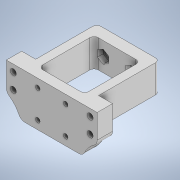
# Autodesk Inventor part: Zcarriage
Saved by Autodesk Inventor 2022 (Build 260153000, 153)
## iProperties
Created: 2022-02-20
Part Number: Zcarriage
Material: Genérico
Document SubType Name: Modeling
Designer: JK
Density: 1 g/cm^3
Appearance: Valor por defecto
Author: JK
Autodesk Inventor part; units mm, degrees
ref_plane "YZ Plane" through (0, 0, 0) normal (1, 0, 0) x (0, 1, 0)
ref_plane "XZ Plane" through (0, 0, 0) normal (0, 1, 0) x (-1, 0, 0)
ref_plane "XY Plane" through (0, 0, 0) normal (0, 0, 1) x (1, 0, 0)
sketch "Boceto1" plane through (0, 0, 0) normal (0, 1, 0) x (-1, 0, 0)
  line L0 (21.032, 35.0057) -> (-23.968, 35.0057)
  line L1 (-23.968, 35.0057) -> (-23.968, 29.0057)
  line L2 (-23.968, 29.0057) -> (21.032, 29.0057)
  line L3 (21.032, 29.0057) -> (21.032, 35.0057)
  line L4 (21.032, -10.7443) -> (-23.968, -10.7443)
  line L5 (-23.968, -10.7443) -> (-23.968, -18.7443)
  line L6 (-23.968, -18.7443) -> (21.032, -18.7443)
  line L7 (21.032, -18.7443) -> (21.032, -10.7443)
  line L8 (21.032, 29.0057) -> (21.032, -18.7443)
  line L9 (-23.968, 29.0057) -> (-23.968, -18.7443)
  line L10 (21.032, 29.0057) -> (21.032, -10.7443)
  line L11 (-23.968, 29.0057) -> (-23.968, -10.7443)
  line L12 (15.032, 29.0057) -> (15.032, -10.7443)
  line L13 (-17.968, 29.0057) -> (-17.968, -10.7443)
  point P0 (0, 0)
  dimension "d0" = 45
  dimension "d1" = 6
  dimension "d3" = 8
  dimension "d4" = 45
  dimension "d7" = 47.75
  dimension "d8" = 6
  dimension "d9" = 6
  constraints: 28 end point, 8 parallel, 6 point on line, 2 horizontal, 2 perpendicular, 1 collinear
  measures "d0" distance of L0.start L0.end
  measures "d1" distance of L2.end L0.start
  measures "d3" distance between parallel lines of L6 L4
  measures "d4" distance of L5.end L6.end
  measures "d7" distance between parallel lines of L6 L2
  measures "d8" distance of L2.end L12.start
  measures "d9" distance of L13.start L1.end
extrude "Extrusión1" add sketch "Boceto1" along normal blind 20 contours L3 L2 L1 L0 | L8 L4 L12 L2 | L2 L13 L4 L9 | L7 L6 L5 L4
sketch "Boceto2" plane through (23.968, 0, -18.7443) normal (0, 0, -1) x (-1, 0, 0)
  circle A0 centre (12.5, 10) radius 2.65
  circle A1 centre (32.5, 10) radius 2.65
  line L0 (0, 0) -> (45, 0) projected
  line L1 (45, 0) -> (45, 20) projected
  point P0 (23.968, 0)
  dimension "d10" = 5.3
  dimension "d11" = 5.3
  dimension "d12" = 20
  dimension "d14" = 10
  dimension "d17" = 12.5
  constraints: 2 centre point, 1 horizontal alignment
  measures "d10" diameter of A0
  measures "d11" diameter of A1
  measures "d12" distance of A1.centre A0.centre
  measures "d14" distance from line of A0.centre L0
  measures "d17" distance from line of L1 A1.centre
extrude "Extrusión2" cut sketch "Boceto2" against normal blind 20
fillet "Empalme1" radius 3 6 edges at (17.968, 10, -10.7443) (-15.032, 10, -10.7443) (17.968, 10, 29.0057) (-15.032, 10, 29.0057) (23.968, 10, -18.7443) (-21.032, 10, -18.7443)
sketch "Boceto3" plane through (-12.032, 0, -10.7443) normal (0, 0, 1) x (1, 0, 0)
  circle A0 centre (23.5, 10) radius 2.65 projected
  circle A1 centre (23.5, 10) radius 4.05
  circle A2 centre (3.5, 10) radius 2.65 projected
  circle A3 centre (3.5, 10) radius 4.05
  line L0 (23.5, 5.3235) -> (19.45, 7.6617)
  line L1 (19.45, 7.6617) -> (19.45, 12.3383)
  line L2 (19.45, 12.3383) -> (23.5, 14.6765)
  line L3 (23.5, 14.6765) -> (27.55, 12.3383)
  line L4 (27.55, 12.3383) -> (27.55, 7.6617)
  line L5 (27.55, 7.6617) -> (23.5, 5.3235)
  line L6 (3.5, 5.3235) -> (-0.55, 7.6617)
  line L7 (-0.55, 7.6617) -> (-0.55, 12.3383)
  line L8 (-0.55, 12.3383) -> (3.5, 14.6765)
  line L9 (3.5, 14.6765) -> (7.55, 12.3383)
  line L10 (7.55, 12.3383) -> (7.55, 7.6617)
  line L11 (7.55, 7.6617) -> (3.5, 5.3235)
  point P0 (12.032, 0)
  dimension "d19" = 8.1
  constraints: 24 end point, 4 coincident, 2 centre point, 2 tangent, 2 vertical alignment, 1 equal radius, 26 other
  measures "d19" diameter of A1
extrude "Extrusión3" cut sketch "Boceto3" along normal blind 20 and the other way blind 4 contours A0 | A1 | L4 L5 A1 | A1 L3 L4 | A1 L2 L3 | L5 L0 A1 | A1 L1 L2 | L0 L1 A1 | A2 | A3 | L10 L11 A3 | A3 L9 L10 | A3 L8 L9 | L11 L6 A3 | A3 L7 L8 | L6 L7 A3
sketch "Boceto4" plane through (0, 0, 0) normal (0, -1, 0) x (1, 0, 0)
  arc A0 (-21.032, -15.7443) -> (-18.032, -18.7443) centre (-18.032, -15.7443) ccw projected
  line L0 (20.968, -18.7443) -> (-18.032, -18.7443) projected
  arc A1 (20.968, -18.7443) -> (23.968, -15.7443) centre (20.968, -15.7443) ccw projected
  line L1 (23.968, 35.0057) -> (23.968, -15.7443) projected
  line L2 (-21.032, 35.0057) -> (23.968, 35.0057) projected
  line L3 (-21.032, -15.7443) -> (-21.032, 35.0057) projected
  arc A2 (-15.032, -7.7443) -> (-12.032, -10.7443) centre (-12.032, -7.7443) ccw projected
  line L4 (-15.032, 26.0057) -> (-15.032, -7.7443) projected
  arc A3 (-12.032, 29.0057) -> (-15.032, 26.0057) centre (-12.032, 26.0057) ccw projected
  line L5 (14.968, 29.0057) -> (-12.032, 29.0057) projected
  arc A4 (17.968, 26.0057) -> (14.968, 29.0057) centre (14.968, 26.0057) ccw projected
  line L6 (17.968, -7.7443) -> (17.968, 26.0057) projected
  arc A5 (14.968, -10.7443) -> (17.968, -7.7443) centre (14.968, -7.7443) ccw projected
  line L7 (-12.032, -10.7443) -> (14.968, -10.7443) projected
  line L8 (-21.032, 35.0057) -> (23.968, 35.0057) projected
  line L9 (23.968, 35.0057) -> (-21.032, 35.0057)
  line L10 (-21.032, 35.0057) -> (-21.032, 29.0057)
  line L11 (-21.032, 29.0057) -> (23.968, 29.0057)
  line L12 (23.968, 29.0057) -> (23.968, 35.0057)
  point P0 (0, 0)
  constraints: 8 end point, 2 parallel, 1 horizontal, 1 perpendicular, 1 point on line
extrude "Extrusión4" add sketch "Boceto4" along normal blind 12 contours L3 L2 L1 L11 L5
chamfer "Chaflán1" distance 12 angle 45 2 edges at (-16.532, 0, 29.0057) (19.468, 0, 29.0057)
sketch "Boceto5" plane through (-21.032, 20, 35.0057) normal (0, 0, 1) x (1, 0, 0)
  circle A0 centre (32.5, -6) radius 1.65
  line L0 (0, 0) -> (45, 0) projected
  line L1 (45, -32) -> (45, 0) projected
  point P0 (21.032, -20)
  dimension "d29" = 3.3
  dimension "d30" = 6
  dimension "d31" = 12.5
  constraints: 1 centre point
  measures "d29" diameter of A0
  measures "d30" distance from line of L0 A0.centre
  measures "d31" distance from line of L1 A0.centre
extrude "Extrusión5" cut sketch "Boceto5" against normal blind 21.5
pattern_linear "Patrón rectangular1" count 2 spacing 20 along (-1, 0, 0) count 2 spacing 20 along (0, -1, 0) of "Extrusión5"
sketch "Boceto6" plane through (-21.032, 20, 35.0057) normal (0, 0, 1) x (1, 0, 0)
  line L0 (-10, 0) -> (55, 0)
  line L1 (55, 0) -> (55, -20)
  line L2 (55, -20) -> (-10, -20)
  line L3 (-10, -20) -> (-10, 0)
  line L4 (0, 0) -> (45, 0) projected
  line L5 (0, -32) -> (0, 0) projected
  line L6 (45, -32) -> (45, 0) projected
  point P0 (21.032, -20)
  point P1 (45, -20)
  point P2 (0, -20)
  dimension "d40" = 10
  dimension "d41" = 10
  dimension "d42" = 20
  constraints: 8 end point, 2 parallel, 1 collinear, 1 horizontal, 1 perpendicular
  measures "d40" distance between parallel lines of L5 L3
  measures "d41" distance between parallel lines of L1 L6
  measures "d42" distance of L2.end L0.start
extrude "Extrusión6" add sketch "Boceto6" against normal blind 10 contours L0 L5 L2 L3 | L0 L1 L2 L6
sketch "Boceto7" plane through (-21.032, -12, 35.0057) normal (0, 0, 1) x (1, 0, 0)
  circle A0 centre (-5, 27) radius 2.15
  line L0 (-10, 32) -> (-10, 12) projected
  line L1 (55, 32) -> (-10, 32) projected
  circle A1 centre (50, 27) radius 2.15
  line L2 (55, 12) -> (55, 32) projected
  circle A2 centre (-5, 16) radius 2.15
  circle A3 centre (50, 16) radius 2.15
  line L3 (45, 12) -> (55, 12) projected
  point P0 (21.032, 12)
  dimension "d45" = 4.3
  dimension "d46" = 5
  dimension "d47" = 5
  dimension "d48" = 5
  dimension "d49" = 5
  dimension "d54" = 11
  constraints: 4 centre point, 3 equal radius, 2 vertical alignment, 1 horizontal alignment
  measures "d45" diameter of A0
  measures "d46" distance from line of L0 A0.centre
  measures "d47" distance from line of L1 A0.centre
  measures "d48" distance from line of L2 A1.centre
  measures "d49" distance from line of L1 A1.centre
  measures "d54" distance of A3.centre A1.centre
extrude "Extrusión7" cut sketch "Boceto7" against normal through all
fillet "Empalme2" radius 20 2 edges at (-21.032, 0, 30.0057) (23.968, 0, 30.0057)
sketch "Boceto8" plane through (-21.032, 20, 25.0057) normal (0, 0, -1) x (-1, 0, 0)
  circle A0 centre (5, -5) radius 2.15 projected
  circle A1 centre (5, -5) radius 3.55
  circle A2 centre (5, -16) radius 2.15 projected
  circle A3 centre (5, -16) radius 3.55
  circle A4 centre (-50, -5) radius 2.15 projected
  circle A5 centre (-50, -5) radius 3.55
  circle A6 centre (-50, -16) radius 2.15 projected
  circle A7 centre (-50, -16) radius 3.55
  line L0 (-50, -0.9008) -> (-46.45, -2.9504)
  line L1 (-46.45, -2.9504) -> (-46.45, -7.0496)
  line L2 (-46.45, -7.0496) -> (-50, -9.0992)
  line L3 (-50, -9.0992) -> (-53.55, -7.0496)
  line L4 (-53.55, -7.0496) -> (-53.55, -2.9504)
  line L5 (-53.55, -2.9504) -> (-50, -0.9008)
  line L6 (-50, -11.9008) -> (-46.45, -13.9504)
  line L7 (-46.45, -13.9504) -> (-46.45, -18.0496)
  line L8 (-46.45, -18.0496) -> (-50, -20.0992)
  line L9 (-50, -20.0992) -> (-53.55, -18.0496)
  line L10 (-53.55, -18.0496) -> (-53.55, -13.9504)
  line L11 (-53.55, -13.9504) -> (-50, -11.9008)
  line L12 (5, -0.9008) -> (8.55, -2.9504)
  line L13 (8.55, -2.9504) -> (8.55, -7.0496)
  line L14 (8.55, -7.0496) -> (5, -9.0992)
  line L15 (5, -9.0992) -> (1.45, -7.0496)
  line L16 (1.45, -7.0496) -> (1.45, -2.9504)
  line L17 (1.45, -2.9504) -> (5, -0.9008)
  line L18 (5, -11.9008) -> (8.55, -13.9504)
  line L19 (8.55, -13.9504) -> (8.55, -18.0496)
  line L20 (8.55, -18.0496) -> (5, -20.0992)
  line L21 (5, -20.0992) -> (1.45, -18.0496)
  line L22 (1.45, -18.0496) -> (1.45, -13.9504)
  line L23 (1.45, -13.9504) -> (5, -11.9008)
  point P0 (-21.032, -20)
  dimension "d55" = 7.1
  constraints: 48 end point, 8 coincident, 4 centre point, 4 tangent, 4 vertical alignment, 3 equal radius, 52 other
  measures "d55" diameter of A5
extrude "Extrusión8" cut sketch "Boceto8" against normal blind 3 contours A0 | A1 | L13 L14 A1 | A1 L12 L13 | A1 L17 L12 | L14 L15 A1 | A1 L16 L17 | L15 L16 A1 | A2 | A3 | L19 L20 A3 | A3 L18 L19 | A3 L23 L18 | L20 L21 A3 | A3 L22 L23 | L21 L22 A3 | A4 | A5 | L1 L2 A5 | A5 L0 L1 | A5 L5 L0 | L2 L3 A5 | A5 L4 L5 | L3 L4 A5 | A6 | A7 | L7 L8 A7 | A7 L6 L7 | A7 L11 L6 | L8 L9 A7 | A7 L10 L11 | L9 L10 A7
sketch "Boceto9" plane through (-31.032, 20, 35.0057) normal (0, 0, 1) x (1, 0, 0)
  circle A0 centre (5, -5) radius 2.15 projected
  circle A1 centre (60, -16) radius 2.15 projected
  circle A2 centre (60, -5) radius 2.15 projected
  circle A3 centre (5, -16) radius 2.15 projected
  circle A4 centre (22.5, -26) radius 1.65 projected
  circle A5 centre (42.5, -26) radius 1.65 projected
  circle A6 centre (22.5, -6) radius 1.65 projected
  circle A7 centre (42.5, -6) radius 1.65 projected
  arc A8 (65, -20) -> (55, -32) centre (74.1445, -37.787) ccw projected
  line L0 (65, -20) -> (65, 0) projected
  line L1 (65, 0) -> (0, 0) projected
  line L2 (0, 0) -> (0, -20) projected
  arc A9 (10, -32) -> (0, -20) centre (-9.1445, -37.787) ccw projected
  line L3 (55, -32) -> (10, -32) projected
  point P0 (31.032, -20)
extrude "Extrusión9" add sketch "Boceto9" along normal blind 1
fillet "Empalme3" radius 5 8 edges at (-31.032, 0, 30.5057) (33.968, 0, 30.5057) (-21.032, -12, 32.5058) (-21.032, -12, 29.0057) (-21.032, -12, 29.0058) (23.968, -12, 32.5058) (23.968, -12, 29.0057) (23.968, -12, 29.0058)
